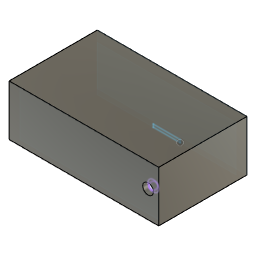
9V Case v1 (Autodesk Fusion 360 design; units mm, degrees)
Autodesk Fusion 360 part; units mm, degrees
note: some values were not read from the file. Set by a fixed rule: which sketch regions a step uses.
sketch "Sketch1" plane through (0, 0, 0) normal (0, 0, 1) x (1, 0, 0)
  line L0 (12, 11) -> (64, 11)
  line L1 (64, 11) -> (64, 40)
  line L2 (64, 40) -> (12, 40)
  line L3 (12, 40) -> (12, 11)
  line L4 (10, 9) -> (66, 9)
  line L5 (66, 9) -> (66, 42)
  line L6 (66, 42) -> (10, 42)
  line L7 (10, 42) -> (10, 9)
  constraint horizontal L0
  constraint vertical L1
  constraint horizontal L2
  constraint vertical L3
  constraint horizontal L4
  constraint vertical L5
  constraint horizontal L6
  constraint vertical L7
extrude "Extrude1" add sketch "Sketch1" along normal blind 19
sketch "Sketch2" plane through (0, 0, 19) normal (0, 0, 1) x (-1, 0, 0)
  line L0 (-12, -11) -> (-12, -40)
  line L1 (-12, -40) -> (-64, -40)
  line L2 (-64, -40) -> (-64, -11)
  line L3 (-64, -11) -> (-12, -11)
  line L4 (-10, -42) -> (-10, -9)
  line L5 (-10, -9) -> (-66, -9)
  line L6 (-66, -9) -> (-66, -42)
  line L7 (-66, -42) -> (-10, -42)
  line L8 (-12, -40) -> (-64, -40)
  line L9 (-64, -40) -> (-64, -11)
  line L10 (-64, -11) -> (-12, -11)
  line L11 (-12, -11) -> (-12, -40)
  constraint horizontal L8
  constraint vertical L9
  constraint horizontal L10
  constraint vertical L11
  constraint coincident L2.end L3.start
  constraint coincident L0.end L1.start
extrude "Extrude2" add sketch "Sketch2" against normal blind 2 contours L0 L1 L2 L3 L8 L9 L10 L11
sketch "Sketch3" plane through (0, 42, 0) normal (0, 1, 0) x (-1, 0, 0)
  line L0 (-66, 0) -> (-10, 0)
  line L1 (-10, 0) -> (-10, 19)
  line L2 (-10, 19) -> (-66, 19)
  line L3 (-66, 19) -> (-66, 0)
sketch "Sketch4" plane through (0, 9, 0) normal (0, -1, 0) x (1, 0, 0)
  line L0 (10, 0) -> (66, 0)
  line L1 (66, 0) -> (66, 19)
  line L2 (66, 19) -> (10, 19)
  line L3 (10, 19) -> (10, 0)
  line L4 (66, 10) -> (64, 10)
  circle A0 centre (62, 10) radius 2
  constraint coincident L1 L4.start
  constraint perpendicular L1 L4
  constraint coincident L4.end A0
hole "Hole2" at (62, 9, 10) direction (0, 1, 0) diameter 4 depth 4 tip angle 118
hole "Hole1" at (63, 9, 10) direction (0, 1, 0) diameter 2 depth 2.2 tip angle 118
sketch "Sketch5" plane through (0, 40, 0) normal (0, -1, 0) x (1, 0, 0)
  line L0 (64, 17) -> (12, 17)
  line L1 (12, 17) -> (12, 0)
  line L2 (12, 0) -> (64, 0)
  line L3 (64, 0) -> (64, 17)
  line L4 (33, 1) -> (43, 1)
  line L5 (33, 1) -> (33, 0)
  line L6 (43, 1) -> (43, 0)
  line L7 (43, 0) -> (33, 0)
  constraint perpendicular L4 L5
  constraint coincident L2 L6.end
  constraint perpendicular L2 L6
  constraint perpendicular L5 L7
extrude "Extrude5" add sketch "Sketch5" along normal blind 2 draft -45 contours L2 L4 L5 L6 L7
extrude "Extrude3" add sketch "Sketch5" along normal blind 3 draft -45 contours L2 L4 L5 L6 L7
sketch "Sketch6" plane through (0, 11, 0) normal (0, 1, 0) x (-1, 0, 0)
  line L0 (-12, 17) -> (-64, 17)
  line L1 (-64, 17) -> (-64, 10)
  line L2 (-64, 10) -> (-64, 0)
  line L3 (-64, 0) -> (-12, 0)
  line L4 (-12, 0) -> (-12, 17)
  circle A0 centre (-62, 10) radius 2
sketch "Sketch7" plane through (38, 11, 8.5) normal (0, 1, 0) x (-1, 0, 0)
  line L0 (5, -7.5) -> (-5, -7.5)
  line L1 (-5, -7.5) -> (-5, -8.5)
  line L2 (-5, -8.5) -> (5, -8.5)
  line L3 (5, -8.5) -> (5, -7.5)
  constraint perpendicular L0 L1
  constraint perpendicular L1 L2
  constraint perpendicular L0 L3
extrude "Extrude4" add sketch "Sketch7" along normal blind 1 draft -45
